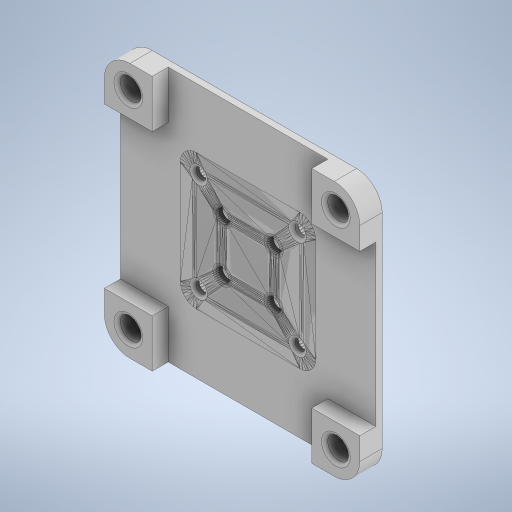
# Autodesk Inventor part: Nema17 Bracket
Saved by Autodesk Inventor 2024 (Build 280153000, 153)
## iProperties
Created: 2025-04-29
Part Number: Nema17 Bracket
Material: Generic
Document SubType Name: Modeling
Designer: Bjarni Heselmans
Density: 1 g/cm^3
Appearance: Default
Author: Bjarni Heselmans
Autodesk Inventor part; units mm, degrees
ref_plane "YZ Plane" through (0, 0, 0) normal (1, 0, 0) x (0, 1, 0)
ref_plane "XZ Plane" through (0, 0, 0) normal (0, 1, 0) x (-1, 0, 0)
ref_plane "XY Plane" through (0, 0, 0) normal (0, 0, 1) x (1, 0, 0)
sketch "Sketch1" plane through (-411.7086, 538.7086, 209.6516) normal (0, 0, 1) x (1, 0, 0)
  line L0 (1224.5086, 477.2914) -> (-401.0914, 477.2914)
  line L1 (-604.2914, 274.0914) -> (-604.2914, -1351.5086)
  line L2 (-401.0914, -1554.7086) -> (1224.5086, -1554.7086)
  line L3 (1427.7086, -1351.5086) -> (1427.7086, 274.0914)
  line L4 (1224.5086, 477.2914) -> (1046.7086, 477.2914)
  line L5 (1046.7086, 477.2914) -> (1046.7086, 96.2914)
  line L6 (1046.7086, 96.2914) -> (1427.7086, 96.2914)
  line L7 (1427.7086, 96.2914) -> (1427.7086, 274.0914)
  line L8 (1224.5086, -1554.7086) -> (1046.7086, -1554.7086)
  line L9 (1046.7086, -1554.7086) -> (1046.7086, -1173.7086)
  line L10 (1046.7086, -1173.7086) -> (1427.7086, -1173.7086)
  line L11 (1427.7086, -1173.7086) -> (1427.7086, -1351.5086)
  circle A0 centre (1237.2086, 286.7914) radius 88.9
  circle A1 centre (1237.2086, -1364.2086) radius 88.9
  arc A2 (1427.7086, 274.0914) -> (1224.5086, 477.2914) centre (1224.5086, 274.0914) ccw
  arc A3 (1224.5086, -1554.7086) -> (1427.7086, -1351.5086) centre (1224.5086, -1351.5086) ccw
  arc A4 (-604.2914, -1351.5086) -> (-401.0914, -1554.7086) centre (-401.0914, -1351.5086) ccw
  arc A5 (-401.0914, 477.2914) -> (-604.2914, 274.0914) centre (-401.0914, 274.0914) ccw
  line L12 (411.7086, -538.7086) -> (1567.4513, -538.7086)
  circle A6 centre (1237.2086, -1364.2086) radius 88.9
  line L13 (411.7086, -538.7086) -> (411.7086, -1318.858)
  circle A7 centre (-413.7914, 286.7914) radius 88.9
  circle A8 centre (-413.7914, -1364.2086) radius 88.9
  line L14 (-223.2914, 477.2914) -> (-223.2914, 96.2914)
  line L15 (-223.2914, 96.2914) -> (-604.2914, 96.2914)
  line L16 (-223.2914, -1554.7086) -> (-223.2914, -1173.7086)
  line L17 (-223.2914, -1173.7086) -> (-604.2914, -1173.7086)
  point P0 (-604.2914, 96.2914)
  point P1 (1427.7086, 96.2914)
  dimension "d0" = 1016
  dimension "d1" = 1016
  dimension "d2" = 1016
  dimension "d3" = 1016
  dimension "d4" = 381
  dimension "d5" = 381
  dimension "d6" = 381
  dimension "d7" = 381
  dimension "d8" = 177.8
  dimension "d9" = 177.8
  dimension "d11" = 203.2
  dimension "d12" = 203.2
  constraints: 36 end point, 9 centre point, 9 symmetric about line, 8 point on circle, 8 tangent, 6 parallel, 4 horizontal, 3 perpendicular, 2 equal radius, 1 vertical, 3 other
  measures "d0" distance from line of L12.start L0
  measures "d1" distance from line of L2 L12.start
  measures "d2" distance from line of L1 L12.start
  measures "d3" distance from line of L3 L12.start
  measures "d4" distance of L6.end L5.end
  measures "d5" distance of L5.end L4.end
  measures "d6" distance of L9.end L10.end
  measures "d7" distance of L8.end L9.end
  measures "d8" diameter of A0
  measures "d9" diameter of A1
  measures "d11" radius of A2
  measures "d12" radius of A3
extrude "Extrusion1" add sketch "Sketch1" along normal blind 127 contours A2 L3 L6 L5 L0 | L14 L15 L1 A5 L0 | L3 A3 L2 L9 L10 | L17 L16 L2 A4 L1
sketch "Sketch2" plane through (-411.7086, 538.7086, 209.6516) normal (0, 0, 1) x (1, 0, 0)
  line L0 (1427.7086, -1351.5086) -> (1427.7086, -1173.7086) projected
  line L1 (-604.2914, 274.0914) -> (-604.2914, 96.2914) projected
  line L2 (1224.5086, -1554.7086) -> (-401.0914, -1554.7086)
  line L3 (-604.2914, -1351.5086) -> (-604.2914, 274.0914)
  line L4 (-401.0914, 477.2914) -> (1224.5086, 477.2914)
  line L5 (1427.7086, 274.0914) -> (1427.7086, -1351.5086)
  arc A0 (1224.5086, -1554.7086) -> (1427.7086, -1351.5086) centre (1224.5086, -1351.5086) ccw
  arc A1 (-604.2914, -1351.5086) -> (-401.0914, -1554.7086) centre (-401.0914, -1351.5086) ccw
  arc A2 (-401.0914, 477.2914) -> (-604.2914, 274.0914) centre (-401.0914, 274.0914) ccw
  arc A3 (1427.7086, 274.0914) -> (1224.5086, 477.2914) centre (1224.5086, 274.0914) ccw
  line L6 (411.7086, -538.7086) -> (614.9086, -538.7086)
  line L7 (614.9086, -538.7086) -> (614.9086, -741.9086)
  line L8 (614.9086, -741.9086) -> (411.7086, -741.9086)
  line L9 (411.7086, -741.9086) -> (411.7086, -538.7086)
  circle A4 centre (614.9086, -741.9086) radius 50.8
  circle A5 centre (208.5086, -741.9086) radius 50.8
  circle A6 centre (614.9086, -335.5086) radius 50.8
  circle A7 centre (208.5086, -335.5086) radius 50.8
  line L10 (411.7086, -538.7086) -> (805.4086, -538.7086)
  line L11 (805.4086, -538.7086) -> (805.4086, -932.4086)
  line L12 (805.4086, -932.4086) -> (411.7086, -932.4086)
  line L13 (411.7086, -932.4086) -> (411.7086, -538.7086)
  circle A8 centre (805.4086, -932.4086) radius 44.45
  circle A9 centre (18.0086, -932.4086) radius 44.45
  circle A10 centre (805.4086, -145.0086) radius 44.45
  circle A11 centre (18.0086, -145.0086) radius 44.45
  line L14 (1107.2821, -735.5586) -> (1116.4989, -735.5586)
  point P0 (-604.2914, -538.7086)
  dimension "d17" = 1016
  dimension "d18" = 1016
  dimension "d19" = 1016
  dimension "d20" = 1016
  dimension "d21" = 203.2
  dimension "d22" = 101.6
  dimension "d23" = 203.2
  dimension "d24" = 203.2
  dimension "d25" = 393.7
  dimension "d26" = 393.7
  dimension "d27" = 88.9
  constraints: 26 end point, 12 centre point, 8 point on circle, 8 tangent, 6 parallel, 6 symmetric about line, 3 equal radius, 3 horizontal, 3 perpendicular, 2 coincident, 1 midpoint, 6 other
  measures "d17" distance from line of L6.start L2
  measures "d18" distance from line of L4 L6.start
  measures "d19" distance of point (-604.291, -538.709) L6.start
  measures "d20" distance from line of L5 L6.start
  measures "d21" radius of A0
  measures "d22" diameter of A4
  measures "d23" distance between parallel lines of L8 L6
  measures "d24" distance between parallel lines of L9 L7
  measures "d25" distance of L11.end L12.end
  measures "d26" distance of L10.end L11.end
  measures "d27" diameter of A8
extrude "Extrusion2" add sketch "Sketch2" against normal blind 50.8 contours A0 L2 A1 L3 L1 A2 L4 A3 L5 L0 | L6 L7 A4 L8 L9 | L10 L11 A8 L12 L13 L8 A4 L7
fillet "Fillet1" radius 25.4 12 edges at (-254, -203.2, 209.6516) (-254, 203.2, 209.6516) (152.4, 203.2, 209.6516) (152.4, -203.2, 209.6516) (-438.15, -393.7, 209.6516) (-438.15, 393.7, 209.6516) (349.25, 393.7, 209.6516) (349.25, -393.7, 209.6516) (736.6, 825.5, 336.6516) (736.6, -825.5, 336.6516) (-914.4, -825.5, 336.6516) (-914.4, 825.5, 336.6516)
body "Solid1"
